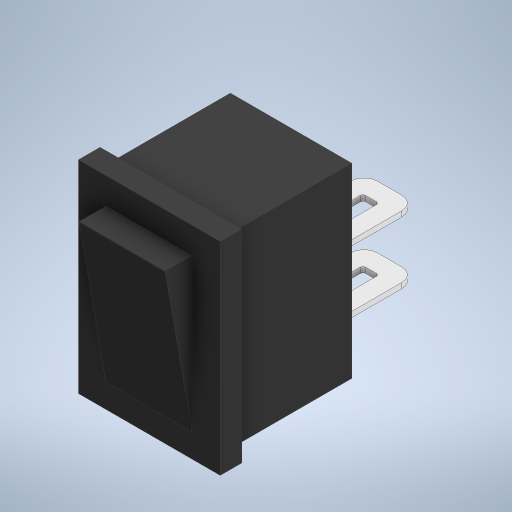
# Autodesk Inventor part: rocker_switch
Saved by Autodesk Inventor 2023 (Build 270158000, 158)
## iProperties
Created: 2023-10-05
Part Number: rocker_switch
Material: Generic
Document SubType Name: Modeling
Designer: mark
Density: 1 g/cm^3
Appearance: Default
Author: mark
Autodesk Inventor part; units mm, degrees
ref_plane "YZ Plane" through (0, 0, 0) normal (1, 0, 0) x (0, 1, 0)
ref_plane "XZ Plane" through (0, 0, 0) normal (0, 1, 0) x (-1, 0, 0)
ref_plane "XY Plane" through (0, 0, 0) normal (0, 0, 1) x (1, 0, 0)
sketch "Sketch1" plane through (0, 0, 0) normal (0, 0, 1) x (1, 0, 0)
  line L0 (0, 0) -> (9, 0)
  line L1 (9, 0) -> (9, 13.8)
  line L2 (9, 13.8) -> (0, 13.8)
  line L3 (0, 13.8) -> (0, 0)
  dimension "d0" = 9
  dimension "d1" = 13.8
  constraints: 8 end point, 2 parallel, 1 horizontal, 1 perpendicular
  measures "d0" distance of L2.end L1.end
  measures "d1" distance of L1.end L0.end
extrude "Extrusion1" add sketch "Sketch1" along normal blind 8.9
sketch "Sketch2" plane through (0, 0, 8.9) normal (0, 0, 1) x (1, 0, 0)
  line L0 (-0.75, 14.4) -> (9.75, 14.4)
  line L1 (9.75, 14.4) -> (9.75, -0.6)
  line L2 (9.75, -0.6) -> (-0.75, -0.6)
  line L3 (-0.75, -0.6) -> (-0.75, 14.4)
  line L4 (9, 13.8) -> (0, 13.8) projected
  line L5 (0, 13.8) -> (0, 0) projected
  dimension "d4" = 10.5
  dimension "d5" = 15
  dimension "d6" = 0.6
  dimension "d7" = 0.75
  constraints: 8 end point, 2 parallel, 1 horizontal, 1 perpendicular
  measures "d4" distance of L0.start L0.end
  measures "d5" distance of L2.end L0.start
  measures "d6" distance between parallel lines of L4 L0
  measures "d7" distance between parallel lines of L3 L5
extrude "Extrusion2" add sketch "Sketch2" along normal blind 1.6
sketch "Sketch3" plane through (0, 0, 10.5) normal (0, 0, 1) x (1, 0, 0)
  line L0 (1.2958, 12.4644) -> (7.672, 12.4644)
  line L1 (7.672, 12.4644) -> (7.672, 1.1518)
  line L2 (7.672, 1.1518) -> (1.2958, 1.1518)
  line L3 (1.2958, 1.1518) -> (1.2958, 12.4644)
  point P0 (0, 0)
  constraints: 8 end point, 2 parallel, 1 horizontal, 1 perpendicular
extrude "Extrusion3" add sketch "Sketch3" along normal blind 2
chamfer "Chamfer1" distance 11.25 angle 10 1 edges at (4.4839, 1.1518, 12.5) measured on face at (4.4839, 1.6518, 12.5)
sketch "Sketch4" plane through (0, 0, 0) normal (0, 0, -1) x (-1, 0, 0)
  line L0 (-6.4, 1.7) -> (-2.6, 1.7)
  line L1 (-2.6, 1.7) -> (-2.6, 1.3)
  line L2 (-2.6, 1.3) -> (-6.4, 1.3)
  line L3 (-6.4, 1.3) -> (-6.4, 1.7)
  line L4 (-9, 0) -> (-9, 13.8) projected
  line L5 (0, 0) -> (-9, 0) projected
  point P0 (-6.4, 1.5)
  dimension "d15" = 3.8
  dimension "d16" = 0.4
  dimension "d17" = 2.6
  dimension "d18" = 1.3
  constraints: 8 end point, 2 parallel, 1 horizontal, 1 midpoint, 1 perpendicular
  measures "d15" distance of L1.end L2.end
  measures "d16" distance of L0.end L1.end
  measures "d17" distance from line of L4 point (-6.4, 1.5)
  measures "d18" distance between parallel lines of L5 L2
extrude "Extrusion4" add sketch "Sketch4" along normal blind 7.3
fillet "Fillet1" radius 1 2 edges at (2.6, 1.5, -7.3) (6.4, 1.5, -7.3)
sketch "Sketch5" plane through (2.6, 1.7, 0) normal (0, 1, 0) x (1, 0, 0)
  line L0 (2.2682, 5.9403) -> (1.4834, 5.9403)
  line L1 (1.2834, 5.7403) -> (1.2834, 3.5404)
  line L2 (1.4834, 3.3404) -> (2.2682, 3.3404)
  line L3 (2.4682, 3.5404) -> (2.4682, 5.7403)
  arc A0 (2.4682, 5.7403) -> (2.2682, 5.9403) centre (2.2682, 5.7403) ccw
  arc A1 (1.4834, 5.9403) -> (1.2834, 5.7403) centre (1.4834, 5.7403) ccw
  arc A2 (2.2682, 3.3404) -> (2.4682, 3.5404) centre (2.2682, 3.5404) ccw
  arc A3 (1.2834, 3.5404) -> (1.4834, 3.3404) centre (1.4834, 3.5404) ccw
  point P0 (-2.6, 0)
  dimension "d22" = 0.2
  constraints: 8 end point, 8 point on circle, 8 tangent, 4 centre point, 3 equal radius, 2 parallel, 1 horizontal, 1 perpendicular
  measures "d22" radius of A0
extrude "Extrusion5" cut sketch "Sketch5" against normal blind 7.3
pattern_linear "Rectangular Pattern1" count 2 spacing 4.6 along (0, 1, 0) of "Extrusion4", "Extrusion5", "Fillet1"
body "Solid1"
